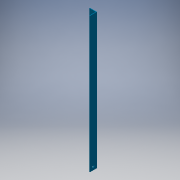
# Autodesk Inventor part: Long Wall Support
Saved by Autodesk Inventor 2017 (Build 210142000, 142)
## iProperties
Created: 2017-01-16
Part Number: Long Wall Support
Material: Aluminum 6061
Document SubType Name: Modeling
Designer: Ben
Density: 2.7 g/cm^3
Appearance: Sky Blue Medium
Mass: 84.6981 g
Surface Area: 404.665 cm^2
Volume: 31.3697 cm^3
Author: Ben
Autodesk Inventor part; units mm, degrees
ref_plane "YZ Plane" through (0, 0, 0) normal (1, 0, 0) x (0, 1, 0)
ref_plane "XZ Plane" through (0, 0, 0) normal (0, 1, 0) x (-1, 0, 0)
ref_plane "XY Plane" through (0, 0, 0) normal (0, 0, 1) x (1, 0, 0)
sketch "Sketch1" plane through (0, 0, 0) normal (0, 1, 0) x (-1, 0, 0)
  line L0 (0, 17.4625) -> (0, 1.5875)
  line L1 (1.5875, 0) -> (17.4625, 0)
  line L2 (17.4625, 0) -> (17.4625, -1.5875)
  line L3 (17.4625, -1.5875) -> (-1.5875, -1.5875)
  line L4 (-1.5875, -1.5875) -> (-1.5875, 17.4625)
  line L5 (-1.5875, 17.4625) -> (0, 17.4625)
  arc A0 (0, 1.5875) -> (1.5875, 0) centre (1.5875, 1.5875) ccw
  point P0 (0, 0)
  dimension "d0" = 1.5875
  dimension "d1" = 19.05
  dimension "d2" = 1.5875
  constraints: 12 end point, 6 perpendicular, 2 point on circle, 2 point on line, 2 tangent, 2 vertical, 1 centre point
  measures "d0" distance of L1.end L2.end
  measures "d1" distance of L2.end L3.end
  measures "d2" radius of A0
extrude "Extrusion1" add sketch "Sketch1" along normal blind 368.3
sketch "Sketch2" plane through (1.5875, 0, -1.5875) normal (0, 0, -1) x (-1, 0, 0)
  line L0 (19.05, 0) -> (0, 0) construction
  line L1 (9.525, 0) -> (9.525, 443.5725) construction
  circle A0 centre (9.525, 9.525) radius 3.175
  point P0 (1.5875, 0)
  dimension "d5" = 6.35
  dimension "d6" = 9.525
  constraints: 2 end point, 1 centre point, 1 midpoint, 1 point on line, 1 vertical
  measures "d5" diameter of A0
  measures "d6" distance from line of L0 A0.centre
extrude "Extrusion2" cut sketch "Sketch2" against normal through all
sketch "Sketch3" plane through (1.5875, 0, 17.4625) normal (1, 0, 0) x (0, 0, -1)
  line L0 (19.05, 0) -> (0, 0) construction
  line L1 (9.525, 0) -> (9.525, 23.4407) construction
  circle A0 centre (9.525, 9.525) radius 3.175
  point P0 (17.4625, 0)
  dimension "d9" = 6.35
  dimension "d10" = 9.525
  constraints: 2 end point, 1 centre point, 1 midpoint, 1 point on line, 1 vertical
  measures "d9" diameter of A0
  measures "d10" distance from line of L0 A0.centre
extrude "Extrusion3" cut sketch "Sketch3" against normal through all
body "Solid1"
